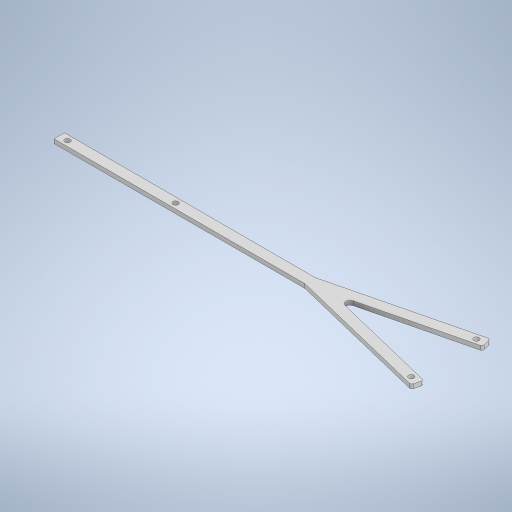
# Autodesk Inventor part: connector
Saved by Autodesk Inventor 2024 (Build 280153000, 153)
## iProperties
Created: 2024-10-22
Part Number: connector
Material: Generic
Document SubType Name: Modeling
Designer: kamil
Density: 1 g/cm^3
Appearance: Default
Author: kamil
Autodesk Inventor part; units mm, degrees
ref_plane "YZ Plane" through (0, 0, 0) normal (1, 0, 0) x (0, 1, 0)
ref_plane "XZ Plane" through (0, 0, 0) normal (0, 1, 0) x (-1, 0, 0)
ref_plane "XY Plane" through (0, 0, 0) normal (0, 0, 1) x (1, 0, 0)
sketch "Sketch1" plane through (0, 0, 0) normal (0, 1, 0) x (-1, 0, 0)
  line L0 (-11.9073, -0.0524) -> (-8.2127, -0.0524) construction
  line L1 (0, 0) -> (-37.2003, 0) construction
  line L2 (-11.9073, -0.0524) -> (-8.256, -0.0524) construction
  line L3 (0, 2.4476) -> (0, 12.311) construction
  line L4 (-46, -2.5) -> (75, -2.5)
  line L5 (75, -2.5) -> (75, 2.5)
  line L6 (75, 2.5) -> (-46, 2.5)
  line L7 (-46, 2.5) -> (-46, -2.5)
  line L8 (-46, 0) -> (75, 0) construction
  line L9 (14.5, -2.5) -> (14.5, 2.5) construction
  circle A0 centre (-110, 15.69) radius 1.3
  circle A1 centre (-110, -15.69) radius 1.3
  line L10 (-46.5953, -2.4281) -> (-45.4047, 2.4281)
  line L11 (-45.4047, 2.4281) -> (-112.3185, 18.8324)
  line L12 (-113.5278, 18.0993) -> (-114.2421, 15.1856)
  line L13 (-113.509, 13.9762) -> (-64.423, 1.9425)
  line L14 (-113.885, 16.6424) -> (-46, 0)
  line L15 (-46.5953, 2.4281) -> (-45.4047, -2.4281)
  line L16 (-45.4047, -2.4281) -> (-112.3185, -18.8324)
  line L17 (-113.5278, -18.0993) -> (-114.2421, -15.1856)
  line L18 (-113.509, -13.9762) -> (-64.423, -1.9425)
  line L19 (-113.885, -16.6424) -> (-46, 0)
  circle A2 centre (71, 0) radius 1.3
  circle A3 centre (19, 0) radius 1.3
  arc A4 (-64.423, -1.9425) -> (-64.423, 1.9425) centre (-64.8992, 0) ccw
  arc A5 (-113.5278, -18.0993) -> (-112.3185, -18.8324) centre (-112.5566, -17.8612) ccw
  arc A6 (-113.509, -13.9762) -> (-114.2421, -15.1856) centre (-113.2709, -14.9475) ccw
  arc A7 (-114.2421, 15.1856) -> (-113.509, 13.9762) centre (-113.2709, 14.9475) ccw
  arc A8 (-112.3185, 18.8324) -> (-113.5278, 18.0993) centre (-112.5566, 17.8612) ccw
  point P0 (-113.2897, 19.0705)
  point P1 (-114.4802, 14.2143)
  point P2 (-113.2897, -19.0705)
  point P3 (-114.4802, -14.2143)
  point P4 (-45.698, 2.5)
  point P5 (-56.4996, 0)
  point P6 (-45.698, -2.5)
  dimension "d10" = 5
  dimension "d12" = 121
  dimension "d13" = 60.5
  dimension "d18" = 2.6
  dimension "d19" = 15.69
  dimension "d21" = 110
  dimension "d24" = 5
  dimension "d25" = 4
  dimension "d26" = 75
  dimension "d29" = 2.6
  dimension "d30" = 4
  dimension "d31" = 2.6
  dimension "d32" = 52
  dimension "d33" = 129
  dimension "d34" = 2
  dimension "d35" = 1
  dimension "d36" = 1
  constraints: 40 end point, 13 point on line, 10 point on circle, 10 tangent, 9 centre point, 6 midpoint, 6 symmetric about line, 4 horizontal, 4 parallel, 2 equal radius, 2 perpendicular, 1 collinear, 1 other
  measures "d10" distance of L4.end L5.end
  measures "d12" distance of L8.end L8.start
  measures "d13" distance between parallel lines of L5 L9
  measures "d18" diameter of A0
  measures "d19" distance from line of L1 A0.centre
  measures "d21" horizontal distance of L1.start A0.centre
  measures "d24" distance of point (-113.29, 19.071) point (-114.48, 14.214)
  measures "d25" distance from line of L12 A0.centre
  measures "d26" distance from line of L1.start L5
  measures "d29" diameter of A2
  measures "d30" distance from line of L5 A2.centre
  measures "d31" diameter of A3
  measures "d32" distance of A3.centre A2.centre
  measures "d33" horizontal distance of A1.centre A3.centre
  measures "d34" radius of A4
  measures "d35" radius of A5
  measures "d36" radius of A7
extrude "Extrusion1" add sketch "Sketch1" along normal blind 2 contours L7 L15 L16 L4 | L4 L16 A5 L17 L19 A1 L7 | L16 L15 L10 L11 L6 L5 L4 | L14 A0 L12 A8 L11 L6 L7 | L7 L6 L11 L10 | L19 A1 L17 A6 L18 A4 L13 A7 L12 L14 A0
sketch "Sketch2" plane through (0, 0, 0) normal (0, -1, 0) x (1, 0, 0)
  line L0 (56, 3.5) -> (56, -3.5)
  line L1 (-75, -2.5) -> (-75, 2.5) projected
  line L2 (-75, 0) -> (62.8992, 0) construction
  arc A0 (64.423, 1.9425) -> (64.423, -1.9425) centre (64.8992, 0) ccw projected
  arc A1 (56, -3.5) -> (56, 3.5) centre (56, 0) ccw
  point P0 (0, 0)
  dimension "d37" = 7
  dimension "d38" = 56
  constraints: 4 end point, 3 point on circle, 2 midpoint, 1 centre point, 1 coincident, 1 horizontal, 1 point on line, 1 vertical
  measures "d37" distance of L0.start L0.end
  measures "d38" distance of point (56, 0) point (0, 0)
revolve "Revolution1" add sketch "Sketch2" angle 180 about axis through (56, 0, 3.5) along (0, 0, -1)
body "Solid1"
